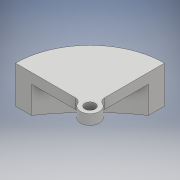
# Autodesk Inventor part: led-holder
Saved by Autodesk Inventor 2018 (Build 220112000, 112)
## iProperties
Created: 2018-03-21
Part Number: led-holder
Material: Generic
Document SubType Name: Modeling
Designer: Matt
Density: 1 g/cm^3
Appearance: Default
Author: Matt
Autodesk Inventor part; units mm, degrees
ref_plane "YZ Plane" through (0, 0, 0) normal (1, 0, 0) x (0, 1, 0)
ref_plane "XZ Plane" through (0, 0, 0) normal (0, 1, 0) x (-1, 0, 0)
sketch "Sketch1" plane through (0, 0, 0) normal (0, 0, 1) x (1, 0, 0)
  arc A0 (0, 22) -> (-22, 0) centre (0, 0) ccw
  arc A1 (0, 17.25) -> (-17.25, 0) centre (38.3744, -38.3744) ccw
  line L0 (0, 17.25) -> (0, 22)
  line L1 (-17.25, 0) -> (-22, 0)
  dimension "d0" = 44
  constraints: 4 end point, 4 point on circle, 2 centre point, 1 coincident, 1 horizontal, 1 vertical
  measures "d0" diameter of A0
ref_plane "Work Plane1" through (0, 0, 16) normal (0, 0, 1) x (1, 0, 0)
extrude "Extrusion3" add sketch "Sketch1" along normal blind 11
sketch "Sketch5" plane through (0, 0, 11) normal (0, 0, 1) x (1, 0, 0)
  arc A0 (0, 17.25) -> (-17.25, 0) centre (38.3744, -38.3744) ccw projected
  line L0 (-4.3084, 0) -> (-17.25, 0)
  line L1 (-2.75, 0) -> (-17.25, 0)
  circle A1 centre (0, 0) radius 1.525
  arc A2 (-2.4943, -1.1579) -> (1.1579, 2.4943) centre (0, 0) ccw
  line L2 (0, 17.25) -> (0, 4.3084)
  line L3 (-17.25, 0) -> (-2.75, 0)
  arc A3 (0, 4.3084) -> (1.1579, 2.4943) centre (2, 4.3084) ccw
  arc A4 (-2.4943, -1.1579) -> (-4.3084, 0) centre (-4.3084, -2) ccw
  point P0 (0, 2.75)
  dimension "d25" = 3.05
  dimension "d26" = 5.5
  dimension "d27" = 2
  constraints: 8 end point, 8 point on circle, 4 centre point, 4 tangent, 2 coincident, 2 point on line, 1 collinear, 1 equal radius, 1 vertical
  measures "d25" diameter of A1
  measures "d26" diameter of A2
  measures "d27" radius of A3
extrude "Extrusion4" add sketch "Sketch5" against normal blind 3
sketch "Sketch6" plane through (0, 0, 0) normal (0, 0, -1) x (-1, 0, 0)
  line L0 (0, 0) -> (15.5563, 15.5563)
  arc A0 (22, 0) -> (0, 22) centre (0, 0) ccw projected
  line L1 (0, 0) -> (22, 0) construction
  circle A1 centre (12.1976, 12.1976) radius 2.8
  dimension "d30" = 45
  dimension "d31" = 5.6
  dimension "d32" = 17.25
  constraints: 4 end point, 1 centre point, 1 equal length, 1 horizontal, 1 point on circle, 1 point on line
  measures "d30" angle of L1 L0
  measures "d31" diameter of A1
  measures "d32" distance of L0.start A1.centre
extrude "Extrusion5" cut sketch "Sketch6" against normal blind 3
body "Solid2"
